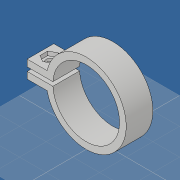
# Autodesk Inventor part: Zyklon_Schelle
Saved by Autodesk Inventor 2019 (Build 230136000, 136)
## iProperties
Created: 2020-09-01
Part Number: Zyklon_Schelle
Material: Generisch
Document SubType Name: Modeling
Designer: Stefan
Mass: 19.4047 g
Surface Area: 102.665 cm^2
Volume: 19.4047 cm^3
Density: 1 g/cm^3
Appearance: Vorgabe
Author: Stefan
Autodesk Inventor part; units mm, degrees
ref_plane "YZ Plane" through (0, 0, 0) normal (1, 0, 0) x (0, 1, 0)
ref_plane "XZ Plane" through (0, 0, 0) normal (0, 1, 0) x (-1, 0, 0)
ref_plane "XY Plane" through (0, 0, 0) normal (0, 0, 1) x (1, 0, 0)
sketch "Skizze1" plane through (0, 0, 0) normal (0, 0, 1) x (1, 0, 0)
  circle A0 centre (0, 0) radius 25 construction
  circle A1 centre (0, 0) radius 30 construction
  line L0 (-24.955, 1.5) -> (-44.2874, 1.5)
  line L1 (-44.2874, 1.5) -> (-44.2874, 6.5)
  line L2 (-44.2874, 6.5) -> (-29.2874, 6.5)
  line L3 (-24.955, -1.5) -> (-44.2874, -1.5)
  line L4 (-44.2874, -1.5) -> (-44.2874, -6.5)
  line L5 (-44.2874, -6.5) -> (-29.2874, -6.5)
  arc A2 (-29.2874, -6.5) -> (-29.2874, 6.5) centre (0, 0) ccw
  arc A3 (-24.955, -1.5) -> (-24.955, 1.5) centre (0, 0) ccw
  line L6 (-59.1448, 0) -> (44.8575, 0) construction
  dimension "d0" = 50
  dimension "d1" = 60
  dimension "d2" = 5
  dimension "d4" = 3
  dimension "d5" = 15
  constraints: 12 end point, 8 point on circle, 4 centre point, 3 perpendicular, 2 coincident, 2 concentric, 2 point on line, 1 collinear, 1 horizontal, 1 parallel, 1 other
  measures "d0" diameter of A0
  measures "d1" diameter of A1
  measures "d2" distance between parallel lines of L0 L2
  measures "d4" distance between parallel lines of L3 L0
  measures "d5" distance of L4.end L5.end
extrude "Extrusion1" add sketch "Skizze1" along normal mid plane 20
sketch "Skizze2" plane through (-44.2874, 6.5, 10) normal (0, 1, 0) x (1, 0, 0)
  line L0 (0, 20) -> (15, 0) construction
  line L1 (15, 20) -> (0, 0) construction
  line L2 (2.5, 12.8868) -> (7.5, 15.7735)
  line L3 (7.5, 15.7735) -> (12.5, 12.8868)
  line L4 (12.5, 12.8868) -> (12.5, 7.1132)
  line L5 (12.5, 7.1132) -> (7.5, 4.2265)
  line L6 (7.5, 4.2265) -> (2.5, 7.1132)
  line L7 (2.5, 7.1132) -> (2.5, 12.8868)
  circle A0 centre (7.5, 10) radius 3.25
  point P0 (44.2874, 10)
  dimension "d8" = 10
  dimension "d9" = 6.5
  constraints: 16 end point, 1 centre point, 1 coincident, 1 midpoint, 1 vertical, 13 other
  measures "d8" distance between parallel lines of L4 L7
  measures "d9" diameter of A0
extrude "Extrusion2" cut sketch "Skizze2" against normal through all contours A0
extrude "Extrusion3" cut sketch "Skizze2" against normal blind 3
